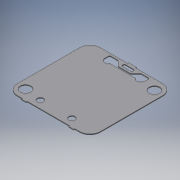
# Autodesk Inventor part: Boden
Saved by Autodesk Inventor 2016 SP2 (Build 200236200, 236)
## iProperties
Created: 2018-06-26
Part Number: Boden
Material: Generisch
Document SubType Name: Modeling
Designer: Nils
Density: 1 g/cm^3
Appearance: Vorgabe
Author: Nils
Autodesk Inventor part; units mm, degrees
ref_plane "YZ Plane" through (0, 0, 0) normal (1, 0, 0) x (0, 1, 0)
ref_plane "XZ Plane" through (0, 0, 0) normal (0, 1, 0) x (-1, 0, 0)
ref_plane "XY Plane" through (0, 0, 0) normal (0, 0, 1) x (1, 0, 0)
sketch "Skizze1" plane through (0, 0, 0) normal (0, 0, 1) x (1, 0, 0)
  line L0 (-3.6885, 36.0919) -> (-3.6885, -23.0081) construction
  arc A0 (-13.6885, -33.0081) -> (-3.6885, -23.0081) centre (-13.6885, -23.0081) ccw construction
  line L1 (-13.6885, -33.0081) -> (-72.7885, -33.0081) construction
  arc A1 (-82.7885, -23.0081) -> (-72.7885, -33.0081) centre (-72.7885, -23.0081) ccw construction
  line L2 (-82.7885, -23.0081) -> (-82.7885, 36.0919) construction
  arc A2 (-72.7885, 46.0919) -> (-82.7885, 36.0919) centre (-72.7885, 36.0919) ccw construction
  line L3 (-72.7885, 46.0919) -> (-13.6885, 46.0919) construction
  arc A3 (-3.6885, 36.0919) -> (-13.6885, 46.0919) centre (-13.6885, 36.0919) ccw construction
  arc A4 (-75.2885, 48.5919) -> (-85.2885, 38.5919) centre (-75.2885, 38.5919) ccw construction
  line L4 (-85.2885, 38.5919) -> (-85.2885, -25.5081) construction
  arc A5 (-85.2885, -25.5081) -> (-75.2885, -35.5081) centre (-75.2885, -25.5081) ccw construction
  line L5 (-75.2885, -35.5081) -> (-11.1885, -35.5081) construction
  arc A6 (-11.1885, -35.5081) -> (-1.1885, -25.5081) centre (-11.1885, -25.5081) ccw construction
  line L6 (-1.1885, -25.5081) -> (-1.1885, 38.5919) construction
  arc A7 (-1.1885, 38.5919) -> (-11.1885, 48.5919) centre (-11.1885, 38.5919) ccw construction
  line L7 (-11.1885, 48.5919) -> (-75.2885, 48.5919) construction
  line L8 (-13.6885, 45.9919) -> (-72.7885, 45.9919)
  arc A8 (-72.7885, 45.9919) -> (-82.6885, 36.0919) centre (-72.7885, 36.0919) ccw
  line L9 (-82.6885, 36.0919) -> (-82.6885, -23.0081)
  arc A9 (-82.6885, -23.0081) -> (-72.7885, -32.9081) centre (-72.7885, -23.0081) ccw
  line L10 (-72.7885, -32.9081) -> (-13.6885, -32.9081)
  arc A10 (-13.6885, -32.9081) -> (-3.7885, -23.0081) centre (-13.6885, -23.0081) ccw
  line L11 (-3.7885, -23.0081) -> (-3.7885, 36.0919)
  arc A11 (-3.7885, 36.0919) -> (-13.6885, 45.9919) centre (-13.6885, 36.0919) ccw
  line L12 (-47.3385, 46.0919) -> (-47.3385, 47.2919) construction
  line L13 (-47.3385, 47.2919) -> (-39.1385, 47.2919) construction
  line L14 (-39.1385, 46.0919) -> (-39.1385, 47.2919) construction
  line L15 (-68.3885, -33.0081) -> (-68.3885, -34.2081) construction
  line L16 (-63.1885, -33.0081) -> (-63.1885, -34.2081) construction
  line L17 (-63.1885, -34.2081) -> (-68.3885, -34.2081) construction
  line L18 (-23.2885, -33.0081) -> (-23.2885, -34.2081) construction
  line L19 (-18.0885, -34.2081) -> (-23.2885, -34.2081) construction
  line L20 (-18.0885, -33.0081) -> (-18.0885, -34.2081) construction
  line L21 (-68.0885, -32.9081) -> (-63.4885, -32.9081)
  line L22 (-63.4885, -32.9081) -> (-63.4885, -33.9081)
  line L23 (-63.4885, -33.9081) -> (-68.0885, -33.9081)
  line L24 (-68.0885, -33.9081) -> (-68.0885, -32.9081)
  line L25 (-22.9885, -32.9081) -> (-18.3885, -32.9081)
  line L26 (-18.3885, -32.9081) -> (-18.3885, -33.9081)
  line L27 (-18.3885, -33.9081) -> (-22.9885, -33.9081)
  line L28 (-22.9885, -33.9081) -> (-22.9885, -32.9081)
  line L29 (-47.0385, 45.9919) -> (-39.4385, 45.9919)
  line L30 (-39.4385, 45.9919) -> (-39.4385, 46.9919)
  line L31 (-39.4385, 46.9919) -> (-47.0385, 46.9919)
  line L32 (-47.0385, 46.9919) -> (-47.0385, 45.9919)
  line L33 (-62.0385, 43.9919) -> (-54.0385, 43.9919)
  line L34 (-54.0385, 43.9919) -> (-49.0385, 38.9919)
  line L35 (-49.0385, 38.9919) -> (-37.0385, 38.9919)
  line L36 (-37.0385, 38.9919) -> (-32.0385, 43.9919)
  line L37 (-32.0385, 43.9919) -> (-24.0385, 43.9919)
  line L38 (-24.0385, 43.9919) -> (-24.0385, 37.4919)
  line L39 (-24.0385, 37.4919) -> (-62.0385, 37.4919)
  line L40 (-62.0385, 37.4919) -> (-62.0385, 43.9919)
  line L41 (-48.0385, 43.9919) -> (-38.0385, 43.9919)
  line L42 (-38.0385, 43.9919) -> (-38.0385, 40.9919)
  line L43 (-38.0385, 40.9919) -> (-48.0385, 40.9919)
  line L44 (-48.0385, 40.9919) -> (-48.0385, 43.9919)
  circle A12 centre (-74.3885, -23.6081) radius 4.075 construction
  circle A13 centre (-12.0885, 36.6919) radius 4.075 construction
  circle A14 centre (-12.0885, 36.6919) radius 5.075
  circle A15 centre (-74.3885, -23.6081) radius 5.075
  arc A16 (-56.277, -27.2081) -> (-60.2001, -27.2081) centre (-58.2385, -25.6581) ccw construction
  arc A17 (-26.277, -27.2081) -> (-30.2001, -27.2081) centre (-28.2385, -25.6581) ccw construction
  arc A18 (-60.1167, 40.3919) -> (-56.3604, 40.3919) centre (-58.2385, 38.7419) ccw construction
  arc A19 (-30.1167, 40.3919) -> (-26.3604, 40.3919) centre (-28.2385, 38.7419) ccw construction
  circle A20 centre (-58.2385, 38.7419) radius 3
  circle A21 centre (-28.2385, 38.7419) radius 3
  circle A22 centre (-58.2385, -25.6581) radius 3
  circle A23 centre (-28.2385, -25.6581) radius 3
  point P0 (0, 0)
  dimension "d0" = 0.1
  dimension "d1" = 0.3
  dimension "d2" = 0.3
  dimension "d3" = 0.3
  dimension "d4" = 0.3
  dimension "d5" = 0.3
  dimension "d6" = 0.3
  dimension "d7" = 0.3
  dimension "d8" = 0.3
  dimension "d9" = 0.3
  dimension "d10" = 135
  dimension "d11" = 1.5
  dimension "d12" = 2
  dimension "d13" = 8
  dimension "d14" = 8
  dimension "d15" = 12
  dimension "d17" = 2
  dimension "d18" = 10
  dimension "d19" = 1
  dimension "d20" = 2
  dimension "d21" = 3
  dimension "d22" = 2
  dimension "d25" = 1
  dimension "d26" = 1
  dimension "d28" = 6
  dimension "d29" = 6
  dimension "d30" = 6
  dimension "d31" = 6
  constraints: 56 end point, 10 centre point, 9 parallel, 8 perpendicular, 8 point on circle, 5 horizontal, 4 coincident, 4 point on line, 7 other
  measures "d0" distance between parallel lines of L3 L8
  measures "d1" distance between parallel lines of L16 L22
  measures "d2" distance between parallel lines of L15 L24
  measures "d3" distance between parallel lines of L17 L23
  measures "d4" distance between parallel lines of L20 L26
  measures "d5" distance between parallel lines of L18 L28
  measures "d6" distance between parallel lines of L19 L27
  measures "d7" distance between parallel lines of L12 L32
  measures "d8" distance between parallel lines of L13 L31
  measures "d9" distance between parallel lines of L14 L30
  measures "d10" angle of L33 L34
  measures "d11" distance between parallel lines of L39 L35
  measures "d12" distance between parallel lines of L8 L33
  measures "d13" distance of L33.start L33.end
  measures "d14" distance of L36.end L37.end
  measures "d15" distance of L34.end L35.end
  measures "d17" distance from line of L34.end L32
  measures "d18" distance of L41.start L41.end
  measures "d19" distance from line of L34.end L44
  measures "d20" distance between parallel lines of L8 L41
  measures "d21" distance between parallel lines of L43 L41
  measures "d22" distance between parallel lines of L35 L43
  measures "d25" radial gap between concentric circles of A13 A14
  measures "d26" radial gap between concentric circles of A12 A15
  measures "d28" diameter of A20
  measures "d29" diameter of A21
  measures "d30" diameter of A22
  measures "d31" diameter of A23
extrude "Extrusion1" add sketch "Skizze1" along normal blind 0.8
fillet "Rundung1" radius 1 12 edges at (-48.0385, 43.9919, 0.4) (-48.0385, 40.9919, 0.4) (-38.0385, 40.9919, 0.4) (-38.0385, 43.9919, 0.4) (-54.0385, 43.9919, 0.4) (-49.0385, 38.9919, 0.4) (-37.0385, 38.9919, 0.4) (-32.0385, 43.9919, 0.4) (-24.0385, 43.9919, 0.4) (-24.0385, 37.4919, 0.4) (-62.0385, 37.4919, 0.4) (-62.0385, 43.9919, 0.4)
equation "\"d1\" = d4"
equation "\"d2\" = d1"
equation "\"d3\" = d1"
equation "\"d5\" = d4"
equation "\"d6\" = d4"
equation "\"d7\" = d9"
equation "\"d8\" = d7"
equation "\"d9\" = d4"
equation "\"d26\" = d25"
equation "\"d29\" = d28"
equation "\"d30\" = d28"
equation "\"d31\" = d28"
